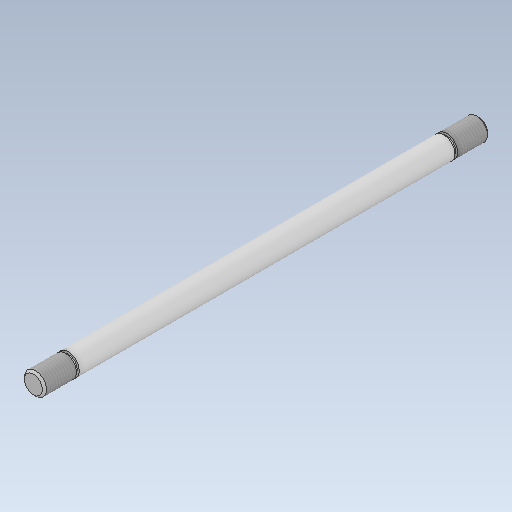
# Autodesk Inventor part: Peça38
Saved by Autodesk Inventor 2021 (Build 250183000, 183)
## iProperties
Category: 41
Created: 2021-07-21
Part Number: Peça38
Material: Genérico
Document SubType Name: Modeling
Designer: Giovanni
Density: 1 g/cm^3
Appearance: Padrão
User Status: 1:2
Author: Giovanni
Keywords: 38
Autodesk Inventor part; units mm, degrees
ref_plane "YZ Plane" through (0, 0, 0) normal (1, 0, 0) x (0, 1, 0)
ref_plane "XZ Plane" through (0, 0, 0) normal (0, 1, 0) x (-1, 0, 0)
ref_plane "XY Plane" through (0, 0, 0) normal (0, 0, 1) x (1, 0, 0)
sketch "Esboço1" plane through (0, 0, 0) normal (0, 0, 1) x (1, 0, 0)
  circle A0 centre (0, 0) radius 8
  dimension "d0" = 16
  constraints: 1 centre point, 1 coincident
  measures "d0" diameter of A0
extrude "Extrusão1" add sketch "Esboço1" along normal mid plane 320
sketch "Esboço2" plane through (0, 0, 0) normal (1, 0, 0) x (0, 1, 0)
  line L0 (8, -160) -> (8, 160) projected
  line L1 (8, -135) -> (6.5, -135)
  line L2 (6.5, -135) -> (6.5, -137)
  line L3 (6.5, -137) -> (8, -137)
  line L4 (8, -137) -> (8, -135)
  line L5 (8, 137) -> (6.5, 137)
  line L6 (6.5, 137) -> (6.5, 135)
  line L7 (6.5, 135) -> (8, 135)
  line L8 (8, 135) -> (8, 137)
  line L9 (8, 160) -> (-8, 160) projected
  line L10 (-8, -160) -> (8, -160) projected
  line L11 (0, 0) -> (0, -160)
  dimension "d3" = 2
  dimension "d4" = 25
  dimension "d5" = 2
  dimension "d6" = 25
  dimension "d7" = 13
  constraints: 18 end point, 4 parallel, 3 point on line, 2 horizontal, 2 perpendicular, 1 midpoint
  measures "d3" distance between parallel lines of L7 L5
  measures "d4" distance between parallel lines of L9 L7
  measures "d5" distance between parallel lines of L3 L1
  measures "d6" distance between parallel lines of L10 L1
  measures "d7" diameter of L2 L11
revolve "Revolução1" cut sketch "Esboço2" angle 360 about axis through (0, 0, 0) along (0, 0, -1)
thread "Rosca1" size "M16x2" class "6g" standard "ANSI Metric M Profile" full length
chamfer "Chanfro1" distance 1.5 angle 45 2 edges at (-8, 0, 160) (-8, 0, -160)
